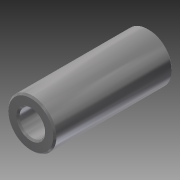
# Autodesk Inventor part: BearingLinearLMUD8
Saved by Autodesk Inventor 2015 (Build 190159000, 159)
## iProperties
Created: 2014-11-30
Part Number: BearingLinearLMUD8
Material: Steel, Mild
Document SubType Name: Modeling
Designer: Jack
Density: 7.85 g/cm^3
Appearance: Semi-Polished
Author: Jack
Autodesk Inventor part; units mm, degrees
ref_plane "YZ Plane" through (0, 0, 0) normal (1, 0, 0) x (0, 1, 0)
ref_plane "XZ Plane" through (0, 0, 0) normal (0, 1, 0) x (-1, 0, 0)
ref_plane "XY Plane" through (0, 0, 0) normal (0, 0, 1) x (1, 0, 0)
sketch "Sketch1" plane through (0, 0, 0) normal (0, 1, 0) x (-1, 0, 0)
  circle A0 centre (0, 0) radius 7.5
  circle A1 centre (0, 0) radius 4
  dimension "d0" = 15
  dimension "d1" = 8
  constraints: 2 centre point, 2 coincident
  measures "d0" diameter of A0
  measures "d1" diameter of A1
extrude "Extrusion1" add sketch "Sketch1" along normal blind 37
chamfer "Chamfer1" distance 0.5 angle 45 4 edges at (7.5, 37, 0) (4, 37, 0) (7.5, 0, 0) (4, 0, 0)
body "Solid1"
